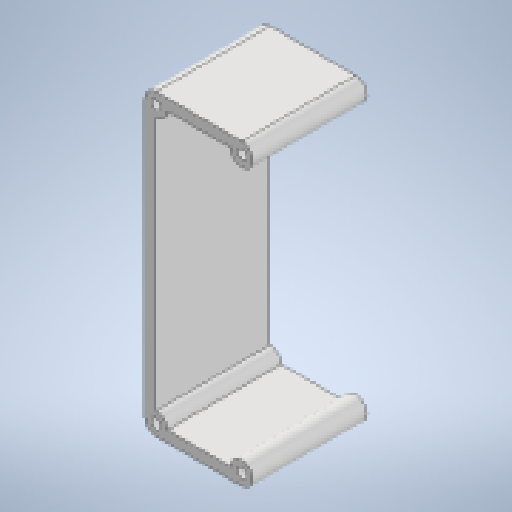
# Autodesk Inventor part: kiban_kakoi
Saved by Autodesk Inventor 2025.1 (Build 291241000, 241)
## iProperties
Created: 2024-09-02
Part Number: kiban_kakoi
Material: 一般
Document SubType Name: Modeling
Designer: right
Density: 1 g/cm^3
Appearance: 既定
Author: right
Autodesk Inventor part; units mm, degrees
ref_plane "YZ Plane" through (0, 0, 0) normal (1, 0, 0) x (0, 1, 0)
ref_plane "XZ Plane" through (0, 0, 0) normal (0, 1, 0) x (-1, 0, 0)
sketch "スケッチ1" plane through (0, 0, 0) normal (0, 0, 1) x (1, 0, 0)
  circle A0 centre (-13.5, 37) radius 1.6 projected
  circle A1 centre (-36.5, 37) radius 1.6 projected
  circle A2 centre (-36.5, -37) radius 1.6 projected
  circle A3 centre (-13.5, -37) radius 1.6 projected
  circle A4 centre (-13.5, 37) radius 1.3
  circle A5 centre (-13.5, 37) radius 3
  circle A6 centre (-36.5, 37) radius 1.3
  circle A7 centre (-36.5, 37) radius 3
  circle A8 centre (-36.5, -37) radius 1.3
  circle A9 centre (-36.5, -37) radius 3
  circle A10 centre (-13.5, -37) radius 1.3
  circle A11 centre (-13.5, -37) radius 3
  line L0 (-13.5, 40) -> (-36.5, 40)
  line L1 (-39.5, 37) -> (-39.5, -37)
  line L2 (-36.5, -40) -> (-13.5, -40)
  line L3 (-16.5, 37) -> (-33.5, 37)
  line L4 (-36.5, 34) -> (-36.5, -34)
  line L5 (-33.5, -37) -> (-16.5, -37)
  point P0 (0, 0)
  dimension "d0" = 2.6
  dimension "d1" = 6
  dimension "d2" = 2.6
  dimension "d3" = 6
  dimension "d4" = 2.6
  dimension "d5" = 6
  dimension "d6" = 2.6
  dimension "d7" = 6
  constraints: 12 end point, 12 point on circle, 8 centre point, 8 coincident, 5 tangent, 3 horizontal alignment, 2 horizontal, 2 vertical alignment
  measures "d0" diameter of A4
  measures "d1" diameter of A5
  measures "d2" diameter of A6
  measures "d3" diameter of A7
  measures "d4" diameter of A8
  measures "d5" diameter of A9
  measures "d6" diameter of A10
  measures "d7" diameter of A11
ref_plane "作業平面1" through (-39.5, -40, 30.5) normal (0, 0, -1) x (0, 1, 0)
extrude "押し出し1" add sketch "スケッチ1" along normal up to surface (30.5 mm away) contours A0 | A1 | A2 | A3 | A5 | A5 L3 A7 L0 | A7 | A7 L4 A9 L1 | A9 | A9 L5 A11 L2 | A11
